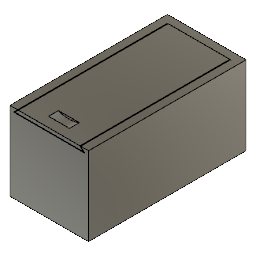
gyakorlati 9 doboz (Autodesk Fusion 360 design; units mm, degrees)
Autodesk Fusion 360 part; units mm, degrees
box "BoxPrimitive1" add length 80 width 40 height 40 placed x (0, 1, 0) y (-1, 0, 0) z (0, 0, 1) at (40, 0, 0) makes body 1 in component "dovoz"
shell "Shell1" thickness 4 removed faces 1 at (13.3333, 26.6667, 40) on bodies 1 in component "dovoz"
sketch "Sketch2" plane through (0, 0, 0) normal (0, -1, 0) x (1, 0, 0) in component "dovoz"
  line L0 (0, 40) -> (0, 0)
  line L1 (0, 0) -> (40, 0)
  line L2 (40, 0) -> (40, 40)
  line L3 (40, 40) -> (0, 40)
  line L4 (36, 40) -> (4, 40)
  line L5 (36, 40) -> (38, 38)
  line L6 (38, 38) -> (36, 40)
  line L7 (20, 40) -> (20, 38) construction
  line L8 (20, 38) -> (38, 38) construction
  line L9 (2, 38) -> (4, 40)
  line L10 (2, 38) -> (38, 38) construction
  line L11 (36, 40) -> (4, 40) construction
  line L12 (2, 38) -> (38, 38)
  line L13 (36, 40) -> (4, 40)
  dimension "d7" = 2.8284
  constraint coincident L4.start L5.start
  constraint midpoint L3 L7.start
  constraint perpendicular L3 L7
  constraint perpendicular L7 L8
  constraint symmetric L4.start L7 L4.end
  constraint symmetric L5.end L7 L9.start
  constraint coincident L4.end L9.end
  measures "d7" distance of L4.start L5.end
extrude "Extrude1" cut sketch "Sketch2" against normal up to surface (76 mm away) contours L3 L4 L5 L6 L9 L12 L13 bodies 1 in component "dovoz"
sketch "Sketch1" plane through (0, 0, 0) normal (0, -1, 0) x (1, 0, 0) in component "fedo"
  line L0 (2, 38) -> (4, 40)
  line L1 (4, 40) -> (0, 40)
  line L2 (0, 40) -> (0, 0)
  line L3 (0, 0) -> (40, 0)
  line L4 (40, 0) -> (40, 40)
  line L5 (40, 40) -> (36, 40)
  line L6 (36, 40) -> (38, 38)
  line L7 (38, 38) -> (2, 38)
  line L8 (4.6036, 40.25) -> (2.6036, 38.25)
  line L9 (2.6036, 38.25) -> (37.3964, 38.25)
  line L10 (35.3964, 40.25) -> (37.3964, 38.25)
  line L11 (35.3964, 40.25) -> (40, 40.25)
  line L12 (4.3533, 39.9998) -> (35.6467, 39.9998)
  constraint coincident L8 L12.start
  constraint coincident L10 L12.end
  constraint horizontal L12
extrude "Extrude1'" add sketch "Sketch1" against normal up to surface (75.99 mm away) separate body contours L8 L9 L10 L12 makes body 2 in component "fedo"
sketch "Sketch2 (2)" plane through (0, 0, 0) normal (0, -1, 0) x (1, 0, 0) in component "fedo"
  line L0 (2.6036, 38.25) -> (37.3964, 38.25)
  line L1 (37.3964, 38.25) -> (35.6467, 39.9998)
  line L2 (35.6467, 39.9998) -> (4.3533, 39.9998)
  line L3 (4.3533, 39.9998) -> (2.6036, 38.25)
  ellipse E0 centre (20, 41) end of major axis (20, 39) minor radius 6.1061
  line L4 (20, 43) -> (20, 39)
  line L5 (13.8939, 41) -> (26.1061, 41)
  constraint perpendicular L2 L4
  constraint coincident E0 L4.start
  constraint coincident E0 L4.end
  constraint coincident E0 L5.start
  constraint coincident E0 L5.end
extrude "Extrude2" cut sketch "Sketch2 (2)" against normal blind 5 from surface at -5 contours L2 E0 L4 | L2 E0 L4 bodies 2 in component "fedo"
component "dovoz" placed x (1, 0, 0) y (0, 1, 0) z (0, 0, 1) at (0, 0, 0)
component "fedo" placed x (1, 0, 0) y (0, 1, 0) z (0, 0, 1) at (0, 0, 0)
